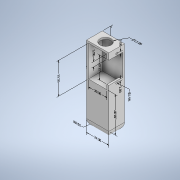
# Autodesk Inventor part: juncao
Saved by Autodesk Inventor 2022.1 (Build 261234000, 234)
## iProperties
Created: 2021-08-02
Part Number: juncao
Material: Generic
Document SubType Name: Modeling
Designer: nakai
Density: 1 g/cm^3
Appearance: Default
Author: nakai
Autodesk Inventor part; units mm, degrees
ref_plane "YZ Plane" through (0, 0, 0) normal (1, 0, 0) x (0, 1, 0)
ref_plane "XZ Plane" through (0, 0, 0) normal (0, 1, 0) x (-1, 0, 0)
ref_plane "XY Plane" through (0, 0, 0) normal (0, 0, 1) x (1, 0, 0)
sketch "Sketch1" plane through (0, 0, 0) normal (0, 0, 1) x (1, 0, 0)
  line L0 (0, 0) -> (24, 0)
  line L1 (24, 0) -> (24, -80)
  line L2 (24, -80) -> (0, -80)
  line L3 (0, -80) -> (0, 0)
  dimension "d0" = 24
  dimension "d1" = 80
  constraints: 8 end point, 2 parallel, 1 horizontal, 1 perpendicular
  measures "d0" distance of L1.end L2.end
  measures "d1" distance of L0.end L1.end
extrude "Extrusion1" add sketch "Sketch1" along normal blind 2
sketch "Sketch2" plane through (0, 0, 2) normal (0, 0, 1) x (1, 0, 0)
  line L0 (0, -80) -> (24, -80) projected
  line L1 (0, 0) -> (2, 0)
  line L2 (2, 0) -> (2, -80)
  line L3 (2, -80) -> (0, -80)
  line L4 (0, -80) -> (0, 0)
  line L5 (24, -80) -> (24, 0) projected
  line L6 (24, 0) -> (22, 0)
  line L7 (22, 0) -> (22, -80)
  line L8 (22, -80) -> (24, -80)
  line L9 (24, -80) -> (24, 0)
  dimension "d4" = 2
  dimension "d5" = 2
  constraints: 16 end point, 4 parallel, 2 horizontal, 2 perpendicular, 2 point on line
  measures "d4" distance of L2.end L3.end
  measures "d5" distance of L8.end L7.end
extrude "Extrusion2" add sketch "Sketch2" along normal blind 15
sketch "Sketch3" plane through (24, -80, 0) normal (1, 0, 0) x (0, 0, -1)
  circle A0 centre (-8.5, 77) radius 1
  circle A1 centre (-8.5, 49.5) radius 1
  line L0 (-17, 0) -> (-17, 80) projected
  line L1 (0, 80) -> (-17, 80) projected
  dimension "d8" = 2
  dimension "d9" = 2
  dimension "d10" = 8.5
  dimension "d11" = 8.5
  dimension "d12" = 27.5
  dimension "d13" = 3
  constraints: 2 centre point
  measures "d8" diameter of A0
  measures "d9" diameter of A1
  measures "d10" distance from line of L0 A0.centre
  measures "d11" distance from line of L0 A1.centre
  measures "d12" distance of A1.centre A0.centre
  measures "d13" distance from line of L1 A0.centre
extrude "Extrusion3" cut sketch "Sketch3" against normal up to surface (2 mm away)
sketch "Sketch4" plane through (24, -80, 0) normal (1, 0, 0) x (0, 0, -1)
  line L0 (-17, 80) -> (-17, 0) projected
  line L1 (-17, 75) -> (-2, 75)
  line L2 (-2, 75) -> (-2, 51.5)
  line L3 (-2, 51.5) -> (-17, 51.5)
  line L4 (-17, 51.5) -> (-17, 75)
  circle A0 centre (-8.5, 77) radius 1 projected
  circle A1 centre (-8.5, 49.5) radius 1 projected
  point P0 (-17, 51.5)
  dimension "d23" = 15
  dimension "d24" = 23.5
  dimension "d25" = 2
  dimension "d26" = 2
  constraints: 8 end point, 2 parallel, 1 horizontal, 1 perpendicular, 1 point on line
  measures "d23" distance of L2.end L3.end
  measures "d24" distance of L1.end L2.end
  measures "d25" distance from line of A0.centre L1
  measures "d26" distance from line of A1.centre L3
extrude "Extrusion4" cut sketch "Sketch4" against normal up to surface (2 mm away) contours L1 L2 L3 L0
sketch "Sketch5" plane through (0, -80, 0) normal (-1, 0, 0) x (0, 0, 1)
  circle A0 centre (8.5, 68.4) radius 2.5
  circle A1 centre (8.5, 77) radius 1 projected
  point P0 (0, 80)
  dimension "d29" = 5
  dimension "d32" = 8.6
  dimension "d33" = 0
  constraints: 1 centre point
  measures "d29" diameter of A0
  measures "d32" distance of A1.centre A0.centre
  measures "d33" horizontal distance of A0.centre A1.centre
extrude "Extrusion5" add sketch "Sketch5" along normal blind 5 contours A0
sketch "Sketch6" plane through (0, -80, 0) normal (0, -1, 0) x (1, 0, 0)
  line L0 (2, 2) -> (22, 2) projected
  line L1 (2, 2) -> (22, 2)
  line L2 (22, 2) -> (22, 17)
  line L3 (22, 17) -> (2, 17)
  line L4 (2, 17) -> (2, 2)
  point P0 (0, 0)
  constraints: 8 end point, 2 parallel, 1 horizontal, 1 perpendicular
extrude "Extrusion6" add sketch "Sketch6" against normal blind 46.5
fillet "Fillet1" radius 8.5 4 edges at (12, -80, 17) (0, -80, 8.5) (12, -80, 0) (24, -80, 8.5)
sketch "Sketch7" plane through (0, 0, 0) normal (0, 1, 0) x (1, 0, 0)
  line L0 (24, 0) -> (24, -17) projected
  line L1 (24, -17) -> (0, -17)
  line L2 (0, -17) -> (0, 0)
  line L3 (0, 0) -> (24, 0)
  line L4 (24, 0) -> (24, -17)
  constraints: 8 end point, 2 parallel, 1 horizontal, 1 perpendicular
extrude "Extrusion7" add sketch "Sketch7" along normal blind 2
sketch "Sketch8" plane through (0, 2, 0) normal (0, 1, 0) x (1, 0, 0)
  circle A0 centre (12, -8.5) radius 6
  line L0 (24, -17) -> (24, 0) projected
  line L1 (0, 0) -> (0, -17) projected
  line L2 (24, 0) -> (0, 0) projected
  dimension "d39" = 12
  dimension "d40" = 12
  dimension "d41" = 24
  dimension "d42" = 17
  dimension "d43" = 8.5
  constraints: 1 centre point
  measures "d39" diameter of A0
  measures "d40" distance from line of L0 A0.centre
  measures "d41" distance between parallel lines of L0 L1
  measures "d42" distance of L1.start L1.end
  measures "d43" distance from line of L2 A0.centre
extrude "Extrusion8" cut sketch "Sketch8" against normal up to surface (2 mm away)
equation "\"d40\" = 0.5 * d41"
equation "\"d43\" = 0.5 * d42"
body "Solid1"
